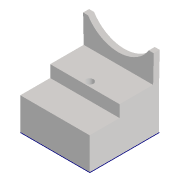
# Autodesk Inventor part: Iris15-mount
Saved by Autodesk Inventor 2021 (Build 250183000, 183)
## iProperties
Created: 2022-05-30
Part Number: Iris15-mount
Material: Generic
Document SubType Name: Modeling
Designer: Nikita
Density: 1 g/cm^3
Appearance: Default
Author: Nikita
Autodesk Inventor part; units mm, degrees
ref_plane "YZ Plane" through (0, 0, 0) normal (1, 0, 0) x (0, 1, 0)
ref_plane "XZ Plane" through (0, 0, 0) normal (0, 1, 0) x (-1, 0, 0)
ref_plane "XY Plane" through (0, 0, 0) normal (0, 0, 1) x (1, 0, 0)
sketch "Sketch1" plane through (0, 0, 0) normal (0, 0, 1) x (1, 0, 0)
  line L0 (29, -29) -> (-29, -29)
  line L1 (-29, -29) -> (-29, 29)
  line L2 (-29, 29) -> (29, 29)
  line L3 (29, 29) -> (29, -29)
  line L4 (29, -29) -> (-29, 29) construction
  line L5 (-29, -29) -> (29, 29) construction
  point P0 (0, 0)
  point P1 (0, 0)
  dimension "d0" = 58
  dimension "d1" = 58
  constraints: 12 end point, 2 midpoint, 2 parallel, 1 coincident, 1 horizontal, 1 perpendicular
  measures "d0" distance of L1.end L2.end
  measures "d1" distance of L0.end L1.end
extrude "Extrusion1" add sketch "Sketch1" along normal blind 36.866
sketch "Sketch2" plane through (0, 0, 36.866) normal (0, 0, 1) x (1, 0, 0)
  line L0 (-29, 29) -> (-29, -29) projected
  line L1 (29, -29) -> (29, 29) projected
  line L2 (-29, -4) -> (29, -4)
  line L3 (29, -4) -> (29, -29)
  line L4 (29, -29) -> (-29, -29)
  line L5 (-29, -29) -> (-29, -4)
  point P0 (0, 0)
  constraints: 8 end point, 2 parallel, 1 horizontal, 1 perpendicular, 1 point on line
extrude "Extrusion2" cut sketch "Sketch2" against normal blind 10
hole "Hole1" at (0, 0, 0) direction (0, 0, 1) diameter 6.5 end through all
sketch "Sketch3" plane through (-29, 29, 0) normal (0, 1, 0) x (1, 0, 0)
  line L0 (0, 0) -> (58, 0) projected
  line L1 (0, 0) -> (0, -36.866) projected
  line L2 (58, -36.866) -> (0, -36.866) projected
  line L3 (58, 0) -> (58, -36.866) projected
  arc A0 (3.645, -60) -> (54.355, -60) centre (29, -75.8) ccw
  line L4 (58, -36.866) -> (58, -26.866) projected
  line L5 (58, -36.866) -> (58.8673, -75.1229)
  line L6 (0, -26.866) -> (0, -36.866) projected
  line L7 (0, -36.866) -> (-0.8673, -76.4771)
  line L8 (58.5245, -60) -> (-0.5065, -60)
  arc A1 (54.355, -60) -> (3.645, -60) centre (29, -75.8) ccw
  point P0 (29, 0)
  dimension "d13" = 59.75
  constraints: 6 end point, 6 point on circle, 4 point on line, 2 centre point, 1 coincident, 1 horizontal, 1 tangent
  measures "d13" diameter of A0
extrude "Extrusion3" add sketch "Sketch3" against normal blind 5 contours L2 L5 L8 A1 L7
body "Solid1"
